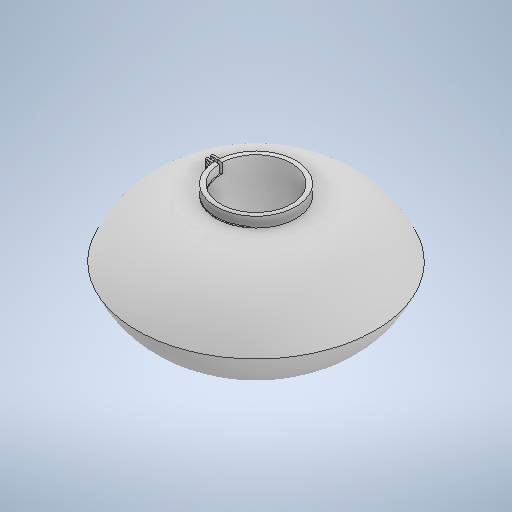
# Autodesk Inventor part: Water Sensor Bouy
Saved by Autodesk Inventor 2025 (Build 290162000, 162)
## iProperties
Created: 2024-06-17
Part Number: Water Sensor Bouy
Material: Generic
Document SubType Name: Modeling
Designer: track
Density: 1 g/cm^3
Appearance: Default
Author: track
## iProperties of the stored document Water Sensor Bouy_3DPrint.ipt
Created: 2024-06-17
Part Number: Water Sensor Bouy_3DPrint
Material: Generic
Document SubType Name: Modeling
Designer: track
Density: 1 g/cm^3
Appearance: Default
Author: track
Autodesk Inventor part; units mm, degrees
sketch "Sketch1" plane through (0, 0, 0) normal (0, 0, 1) x (1, 0, 0)
  line L0 (0, 0) -> (0, 76.2)
  line L1 (31.226, 0) -> (31.226, 101.6)
  line L2 (31.226, 50.8) -> (104.886, 50.8)
  arc A0 (104.886, 50.8) -> (31.226, 101.6) centre (31.226, 22.7965) ccw
  arc A1 (31.226, 0) -> (104.886, 50.8) centre (31.226, 78.8035) ccw
  line L3 (32.226, 100.5936) -> (32.226, 1.0064)
  arc A2 (32.226, 1.0064) -> (103.8152, 50.8) centre (31.226, 78.8035) ccw
  arc A3 (103.8152, 50.8) -> (32.226, 100.5936) centre (31.226, 22.7965) ccw
  point P0 (31.226, 25.4)
  point P1 (88.0908, 24.2472)
  point P2 (32.226, 31.75)
  point P3 (86.773, 24.325)
  point P4 (32.226, 50.8)
  dimension "d0" = 101.6
  dimension "d1" = 31.226
  dimension "d2" = 50.8
  dimension "d3" = 0
  dimension "d4" = 73.66
  dimension "d24" = 78.8035
  dimension "d33" = 1
  constraints: 10 point on circle, 8 end point, 4 centre point, 4 point on line, 2 vertical, 1 horizontal, 1 midpoint, 2 other
  measures "d0" distance of L1.start L1.end
  measures "d1" distance between parallel lines of L1 L0
  measures "d2" distance from line of L1.end L2
  measures "d3" vertical distance of L0.start L1.start
  measures "d4" distance of L2.start L2.end
  measures "d24" radius of A0
  measures "d33" distance between parallel lines of L1 L3
revolve "Revolution1" add sketch "Sketch1" angle 360 about axis through (0, 0, 0) along (0, 1, 0) contours L1 L2 L3 A2 A1 | L1 A0 L2 A3 L3
sketch "Sketch6" plane through (0, 0, 0) normal (0, 0, 1) x (1, 0, 0)
  arc A0 (104.886, 50.8) -> (31.226, 101.6) centre (31.226, 22.7965) ccw projected
  line L0 (31.226, 101.6) -> (-31.226, 101.6) projected
  arc A1 (99.1182, 62.8044) -> (31.226, 101.6) centre (31.226, 22.7965) ccw
  line L1 (65.4318, 93.7892) -> (35.3304, 50.8)
  line L2 (103.8152, 50.8) -> (-103.8152, 50.8) projected
  point P0 (0, 0)
  dimension "d34" = 55
  dimension "d35" = 12.7
  constraints: 4 point on circle, 2 end point, 1 centre point, 1 concentric, 1 point on line
  measures "d34" angle of L2 L1
  measures "d35" distance from line of A0.centre L1
ref_plane "Work Plane4" through (65.4318, 93.7892, 0) normal (0.4341, 0.9009, 0) x (-0.9009, 0.4341, 0)
sketch "Sketch26" plane through (0, 0, 0) normal (0, 1, 0) x (-1, 0, 0)
  line L0 (0, 0) -> (-13.716, 0)
  circle A0 centre (-63.5, 0) radius 3.175
  dimension "d142" = 6.35
  dimension "d143" = 63.5
  constraints: 2 end point, 1 centre point, 1 horizontal, 1 point on line
  measures "d142" diameter of A0
  measures "d143" distance of L0.start A0.centre
extrude "Extrusion17" cut sketch "Sketch26" along normal blind 25
pattern_circular "Circular Pattern5" count 3 over 360 about axis through (0, 78.8035, 0) along (0, 1, 0) of "Extrusion17"
ref_plane "Work Plane7" through (0, 101.6, 0) normal (0, 1, 0) x (-1, 0, 0)
sketch "Sketch30" plane through (0, 101.6, 0) normal (0, 1, 0) x (-1, 0, 0)
  circle A0 centre (0, 0) radius 31.226
  circle A1 centre (0, 0) radius 31.226 projected
  circle A2 centre (0, 0) radius 31.226
  circle A3 centre (0, 0) radius 35.226
  dimension "d161" = 4
  constraints: 3 centre point, 3 coincident, 2 concentric
  measures "d161" radial gap between concentric circles of A3 A0
extrude "Extrusion21" add sketch "Sketch30" along normal blind 8.89 and the other way blind 2
ref_plane "Work Plane8" through (-35.226, 101.6, 0) normal (1, 0, 0) x (0, 1, 0)
sketch "Sketch32" plane through (-35.226, 101.6, 0) normal (1, 0, 0) x (0, 1, 0)
  line L0 (8.89, 31.226) -> (8.89, -31.226) projected
  line L1 (8.89, -3.27) -> (0, -3.27)
  line L2 (0, -3.27) -> (0, -1.27)
  line L3 (0, -1.27) -> (8.89, -1.27)
  line L4 (8.89, -1.27) -> (8.89, -3.27)
  line L5 (0, 1.27) -> (8.89, 1.27)
  line L6 (8.89, 1.27) -> (8.89, 3.27)
  line L7 (8.89, 3.27) -> (0, 3.27)
  line L8 (0, 3.27) -> (0, 1.27)
  line L9 (8.89, 0) -> (0.002, 0)
  line L10 (-0.1016, 35.226) -> (-0.1016, -35.226) projected
  point P0 (-101.6, 0)
  point P1 (8.89, 3.27)
  dimension "d167" = 8.89
  dimension "d168" = 2.54
  dimension "d169" = 2
  constraints: 18 end point, 5 parallel, 3 point on line, 2 horizontal, 2 perpendicular, 1 midpoint, 2 other
  measures "d167" distance between parallel lines of L0 L2
  measures "d168" distance between parallel lines of L5 L3
  measures "d169" distance of L7.end L5.start
extrude "Extrusion22" add sketch "Sketch32" against normal blind 6.35
sketch "Sketch34" plane through (-41.576, 101.6, 0) normal (-1, 0, 0) x (0, 0, 1)
  line L0 (-1.27, 8.89) -> (-1.27, 0) projected
  line L1 (1.27, 8.89) -> (1.27, 0) projected
  line L2 (-1.27, 8.89) -> (1.27, 8.89)
  line L3 (1.27, 8.89) -> (1.27, 1)
  line L4 (1.27, 0) -> (-1.27, 0)
  line L5 (-1.27, 0) -> (-1.27, 8.89)
  line L6 (35.226, -0.1016) -> (35.226, 8.89) projected
  line L7 (1.27, 1) -> (35.226, 1)
  line L8 (35.226, 1) -> (35.226, 0)
  line L9 (35.226, 0) -> (1.27, 0)
  point P0 (0, -101.6)
  point P1 (35.226, 1)
  point P2 (1.27, 1)
  dimension "d172" = 1
  constraints: 14 end point, 3 parallel, 2 horizontal, 2 perpendicular, 2 point on line
  measures "d172" distance between parallel lines of L9 L7
extrude "Extrusion23" cut sketch "Sketch34" against normal blind 63.5
sketch "Sketch35" plane through (-41.576, 110.49, 3.27) normal (0, 0, 1) x (1, 0, 0)
  line L0 (6.35, 0) -> (0, 0) projected
  line L1 (2.54, 0) -> (2.54, -7.89)
  line L2 (0, -7.89) -> (6.35, -7.89) projected
  line L3 (0, -7.89) -> (0, 0) projected
  circle A0 centre (2.54, -1.905) radius 1.27
  circle A1 centre (2.54, -5.985) radius 1.27
  point P0 (41.576, -110.49)
  dimension "d175" = 2.54
  dimension "d176" = 2.54
  dimension "d177" = 2.54
  dimension "d178" = 1.905
  dimension "d179" = 1.905
  constraints: 4 point on line, 2 centre point, 2 end point, 1 vertical
  measures "d175" distance between parallel lines of L3 L1
  measures "d176" diameter of A0
  measures "d177" diameter of A1
  measures "d178" distance from line of L0 A0.centre
  measures "d179" distance from line of L2 A1.centre
extrude "Extrusion24" cut sketch "Sketch35" against normal up to surface (6.54 mm away) contours A0 L1 | L1 A0 | A1 L1 | L1 A1
body "Solid1"
